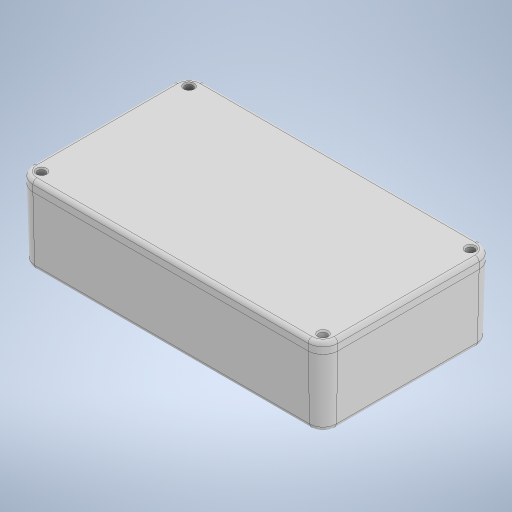
# Autodesk Inventor part: RSpro.Al_DieCast_114x63x30
Saved by Autodesk Inventor 2023 (Build 270158030, 158C)
## iProperties
Created: 2022-11-09
Part Number: RSpro.Al_DieCast_114x63x30
Material: Generic
Document SubType Name: Modeling
Designer: Imogen Heard
Density: 1 g/cm^3
Appearance: Default
Author: Imogen Heard
Autodesk Inventor part; units mm, degrees
ref_plane "YZ Plane" through (0, 0, 0) normal (1, 0, 0) x (0, 1, 0)
ref_plane "XZ Plane" through (0, 0, 0) normal (0, 1, 0) x (-1, 0, 0)
sketch "Sketch1" plane through (0, 0, 0) normal (0, 1, 0) x (-1, 0, 0)
  line L0 (-5, -63.6) -> (-109.5, -63.6)
  line L1 (-114.5, -58.6) -> (-114.5, -5)
  line L2 (-109.5, 0) -> (-5, 0)
  line L3 (0, -5) -> (0, -58.6)
  arc A0 (-5, -63.6) -> (0, -58.6) centre (-5, -58.6) ccw
  arc A1 (-114.5, -58.6) -> (-109.5, -63.6) centre (-109.5, -58.6) ccw
  arc A2 (-109.5, 0) -> (-114.5, -5) centre (-109.5, -5) ccw
  arc A3 (0, -5) -> (-5, 0) centre (-5, -5) ccw
  point P0 (0, 0)
  point P1 (0, 0)
  dimension "d0" = 114.5
  dimension "d1" = 63.6
  dimension "d2" = 5
  constraints: 8 end point, 8 point on circle, 8 tangent, 4 centre point, 3 equal radius, 2 parallel, 2 point on line, 1 coincident, 1 horizontal, 1 perpendicular
  measures "d0" distance between parallel lines of L1 L3
  measures "d1" distance between parallel lines of L0 L2
  measures "d2" radius of A0
extrude "Extrusion1" add sketch "Sketch1" along normal blind 26.3 draft 1.5
sketch "Sketch2" plane through (0, 26.3, 0) normal (0, 1, 0) x (1, 0, 0)
  line L0 (4.8113, 62.7887) -> (109.6887, 62.7887)
  line L1 (113.6887, 58.7887) -> (113.6887, 4.8113)
  line L2 (109.6887, 0.8113) -> (4.8113, 0.8113)
  line L3 (0.8113, 4.8113) -> (0.8113, 58.7887)
  line L4 (115.1887, 58.6) -> (115.1887, 5) projected
  line L5 (109.5, -0.6887) -> (5, -0.6887) projected
  line L6 (5, 64.2887) -> (109.5, 64.2887) projected
  line L7 (-0.6887, 5) -> (-0.6887, 58.6) projected
  arc A0 (4.8113, 62.7887) -> (0.8113, 58.7887) centre (4.8113, 58.7887) ccw
  arc A1 (113.6887, 58.7887) -> (109.6887, 62.7887) centre (109.6887, 58.7887) ccw
  arc A2 (109.6887, 0.8113) -> (113.6887, 4.8113) centre (109.6887, 4.8113) ccw
  arc A3 (0.8113, 4.8113) -> (4.8113, 0.8113) centre (4.8113, 4.8113) ccw
  point P0 (0, 0)
  point P1 (115.1887, 31.8)
  point P2 (57.25, 0.8113)
  dimension "d12" = 1.5
  dimension "d13" = 1.5
  dimension "d14" = 1.5
  dimension "d15" = 1.5
  dimension "d16" = 4
  dimension "d20" = 4
  dimension "d21" = 4
  constraints: 8 end point, 8 point on circle, 8 tangent, 4 centre point, 3 equal radius, 2 midpoint, 2 parallel, 1 horizontal, 1 perpendicular
  measures "d12" distance from line of point (115.189, 31.8) L1
  measures "d13" distance from line of L5 point (57.25, 0.811)
  measures "d14" distance between parallel lines of L6 L0
  measures "d15" distance between parallel lines of L7 L3
  measures "d16" radius of A0
  measures "d20" radius of A3
  measures "d21" radius of A1
ref_plane "Work Plane1" through (0, 1.5, 0) normal (0, -1, 0) x (1, 0, 0)
extrude "Extrusion2" cut sketch "Sketch2" against normal up to surface (24.8 mm away) draft -1.5
sketch "Sketch3" plane through (4.8113, 1.5, -1.4607) normal (0, 1, 0) x (1, 0, 0)
  circle A0 centre (-1.0113, 2.3393) radius 2.65
  circle A1 centre (-1.0113, 58.3393) radius 2.65
  circle A2 centre (105.8887, 2.3393) radius 2.65
  circle A3 centre (105.8887, 58.3393) radius 2.65
  line L0 (-4.8113, 57.1393) -> (-4.8113, 3.5393) projected
  line L1 (0.1887, -1.4607) -> (104.6887, -1.4607) projected
  line L2 (104.6887, 62.1393) -> (0.1887, 62.1393) projected
  line L3 (109.6887, 3.5393) -> (109.6887, 57.1393) projected
  point P0 (-4.8113, -1.4607)
  dimension "d22" = 5.3
  dimension "d23" = 3.8
  dimension "d24" = 3.8
  dimension "d25" = 3.8
  dimension "d26" = 3.8
  constraints: 4 centre point, 3 equal radius, 2 horizontal alignment, 2 vertical alignment
  measures "d22" diameter of A0
  measures "d23" distance from line of L0 A0.centre
  measures "d24" distance from line of L1 A0.centre
  measures "d25" distance from line of L2 A1.centre
  measures "d26" distance from line of L3 A2.centre
extrude "Extrusion3" add sketch "Sketch3" along normal up to surface (24.8 mm away)
fillet "Fillet1" radius 1.5 8 edges at (4.9295, 3.7123, -1.4028) (1.4028, 3.7123, -4.9295) (1.4028, 3.7123, -58.6705) (4.9295, 3.7123, -62.1972) (109.5705, 3.7123, -1.4028) (113.0972, 3.7123, -4.9295) (113.0972, 3.7123, -58.6705) (109.5705, 3.7123, -62.1972)
sketch "Sketch4" plane through (0, 26.3, 0) normal (0, 1, 0) x (1, 0, 0)
  circle A0 centre (3.8, 3.8) radius 1.5
  circle A1 centre (3.8, 59.8) radius 1.5
  circle A2 centre (110.7, 3.8) radius 1.5
  circle A3 centre (110.7, 59.8) radius 1.5
  arc A4 (108.2262, 60.7503) -> (111.6503, 57.3262) centre (110.7, 59.8) ccw projected
  arc A5 (111.6503, 6.2738) -> (108.2262, 2.8497) centre (110.7, 3.8) ccw projected
  arc A6 (2.8497, 57.3262) -> (6.2738, 60.7503) centre (3.8, 59.8) ccw projected
  arc A7 (6.2738, 2.8497) -> (2.8497, 6.2738) centre (3.8, 3.8) ccw projected
  point P0 (0, 0)
  point P1 (111.686, 56.2611)
  point P2 (107.1611, 60.786)
  point P3 (107.1611, 2.814)
  point P4 (111.686, 7.3389)
  point P5 (7.3389, 60.786)
  point P6 (2.814, 56.2611)
  point P7 (2.814, 7.3389)
  point P8 (7.3389, 2.814)
  dimension "d30" = 3
  constraints: 4 centre point, 4 concentric, 3 equal radius
  measures "d30" diameter of A0
fillet "Fillet2" radius 2 8 edges at (113.0355, 0, -62.1355) (57.25, 0, -63.6) (1.4645, 0, -62.1355) (0, 0, -31.8) (1.4645, 0, -1.4645) (57.25, 0, 0) (113.0355, 0, -1.4645) (114.5, 0, -31.8)
hole "Hole1" at (110.7, 26.3, -59.8) at (3.8, 26.3, -59.8) at (3.8, 26.3, -3.8) at (110.7, 26.3, -3.8) direction (0, -1, 0) diameter 2.85 depth 20 tip angle 118 thread size "M3.5x0.6" class "6H" standard "ISO Metric profile"
sketch "Sketch5" plane through (0, 26.3, 0) normal (0, 1, 0) x (1, 0, 0)
  line L0 (4.9813, 64.2887) -> (109.5187, 64.2887)
  line L1 (115.1887, 58.6187) -> (115.1887, 4.9813)
  line L2 (109.5187, -0.6887) -> (4.9813, -0.6887)
  line L3 (-0.6887, 4.9813) -> (-0.6887, 58.6187)
  arc A0 (4.9813, 64.2887) -> (-0.6887, 58.6187) centre (4.9813, 58.6187) ccw
  arc A1 (115.1887, 58.6187) -> (109.5187, 64.2887) centre (109.5187, 58.6187) ccw
  arc A2 (109.5187, -0.6887) -> (115.1887, 4.9813) centre (109.5187, 4.9813) ccw
  arc A3 (-0.6887, 4.9813) -> (4.9813, -0.6887) centre (4.9813, 4.9813) ccw
  point P0 (0, 0)
  point P1 (-0.6887, 64.2887)
  point P2 (115.1887, -0.6887)
  point P3 (-0.6887, -0.6887)
  point P4 (5, 64.2887)
  point P5 (5, -0.6887)
  point P6 (115.1887, 5)
  point P7 (-0.6887, 5)
  dimension "d39" = 5.67
  constraints: 8 end point, 8 point on circle, 8 tangent, 6 point on line, 4 centre point, 3 equal radius, 2 horizontal alignment, 2 parallel, 2 vertical alignment, 1 horizontal, 1 perpendicular
  measures "d39" radius of A0
extrude "Extrusion4" add sketch "Sketch5" along normal blind 4 separate body
fillet "Fillet3" radius 1.5 8 edges at (113.528, 30.3, -0.972) (115.1887, 30.3, -31.8) (113.528, 30.3, -62.628) (57.25, 30.3, -64.2887) (0.972, 30.3, -62.628) (-0.6887, 30.3, -31.8) (0.972, 30.3, -0.972) (57.25, 30.3, 0.6887)
sketch "Sketch6" plane through (0, 30.3, 0) normal (0, 1, 0) x (1, 0, 0)
  circle A0 centre (3.8, 59.8) radius 1.5
  circle A1 centre (110.7, 59.8) radius 1.5
  circle A2 centre (3.8, 3.8) radius 1.5
  circle A3 centre (110.7, 3.8) radius 1.5
  circle A4 centre (3.8, 59.8) radius 1.425 projected
  circle A5 centre (110.7, 59.8) radius 1.425 projected
  circle A6 centre (110.7, 3.8) radius 1.425 projected
  circle A7 centre (3.8, 3.8) radius 1.425 projected
  point P0 (0, 0)
  dimension "d43" = 3
  constraints: 4 centre point, 4 concentric, 3 equal radius
  measures "d43" diameter of A0
hole "Hole2" at (3.8, 30.3, -59.8) at (110.7, 30.3, -59.8) at (110.7, 30.3, -3.8) at (3.8, 30.3, -3.8) direction (0, -1, 0) diameter 3 depth 4 tip angle 118 countersink diameter 4 countersink angle 90 bodies 2
sketch "Sketch7" plane through (0, 26.3, 0) normal (0, -1, 0) x (1, 0, 0)
  line L0 (113.1887, -10.8113) -> (113.1887, -52.7887)
  line L1 (103.6887, -62.2887) -> (10.8113, -62.2887)
  line L2 (1.3113, -52.7887) -> (1.3113, -10.8113)
  line L3 (10.8113, -2.3113) -> (103.6887, -2.3113)
  line L4 (111.6887, -10.8113) -> (111.6887, -52.7887)
  line L5 (103.6887, -61.2887) -> (10.8113, -61.2887)
  line L6 (2.3113, -52.7887) -> (2.3113, -10.8113)
  line L7 (106.8264, -0.8113) -> (7.6736, -0.8113) projected
  line L8 (7.6736, -62.7887) -> (106.8264, -62.7887) projected
  line L9 (0.8113, -7.6736) -> (0.8113, -55.9264) projected
  line L10 (113.6887, -55.9264) -> (113.6887, -7.6736) projected
  arc A0 (108.2262, -2.8497) -> (111.6503, -6.2738) centre (110.7, -3.8) ccw projected
  line L11 (10.8113, -1.3113) -> (103.6887, -1.3113)
  line L12 (113.1887, -10.8113) -> (111.6887, -10.8113)
  line L13 (103.6887, -2.3113) -> (103.6887, -1.3113)
  line L14 (103.6887, -62.2887) -> (103.6887, -61.2887)
  line L15 (111.6887, -52.7887) -> (113.6887, -52.7887)
  line L16 (10.8113, -61.2887) -> (10.8113, -62.2887)
  line L17 (10.8113, -1.3113) -> (10.8113, -2.3113)
  line L18 (2.3113, -10.8113) -> (1.3113, -10.8113)
  line L19 (1.3113, -52.7887) -> (2.3113, -52.7887)
  point P0 (0, 0)
  point P1 (103.6887, -52.7887)
  point P2 (7.8641, -10.8113)
  point P3 (103.6887, -1.8113)
  point P4 (1.8113, -52.7887)
  point P5 (112.6887, -52.7887)
  point P6 (10.8113, -1.8113)
  point P7 (10.8113, -61.7887)
  point P8 (7.8641, -62.1393)
  point P9 (103.6887, -61.7887)
  point P10 (1.8113, -10.8113)
  point P11 (112.4387, -10.8113)
  dimension "d52" = 0.5
  dimension "d53" = 0.5
  dimension "d54" = 0.5
  dimension "d55" = 1.5
  dimension "d56" = 1.5
  dimension "d57" = 1.5
  dimension "d58" = 1.5
  dimension "d60" = 0.5
  dimension "d62" = 10
  dimension "d63" = 10
  dimension "d64" = 10
  dimension "d65" = 10
  constraints: 32 end point, 8 midpoint, 5 horizontal alignment, 4 parallel, 4 vertical alignment, 2 horizontal, 2 perpendicular, 2 point on line
  measures "d52" distance between parallel lines of L8 L1
  measures "d53" distance between parallel lines of L9 L2
  measures "d54" distance between parallel lines of L10 L0
  measures "d55" distance between parallel lines of L0 L4
  measures "d56" distance between parallel lines of L7 L3
  measures "d57" distance between parallel lines of L6 L9
  measures "d58" distance between parallel lines of L5 L8
  measures "d60" distance between parallel lines of L11 L7
  measures "d62" distance between parallel lines of L7 L12
  measures "d63" distance between parallel lines of L10 L13
  measures "d64" distance between parallel lines of L8 L15
  measures "d65" distance between parallel lines of L9 L16
extrude "Extrusion5" add sketch "Sketch7" along normal blind 2.5 bodies 2
sketch "Sketch8" plane through (0, 26.3, 0) normal (0, -1, 0) x (1, 0, 0)
  line L0 (10.8113, -2.3113) -> (103.6887, -2.3113)
  line L1 (111.6887, -10.8113) -> (111.6887, -52.7887)
  line L2 (103.6887, -61.2887) -> (10.8113, -61.2887)
  line L3 (2.3113, -52.7887) -> (2.3113, -10.8113)
  line L4 (2.3113, -10.8113) -> (1.3113, -10.8113) projected
  arc A0 (2.3113, -10.8113) -> (10.8113, -2.3113) centre (1.8245, -1.8245) ccw
  arc A1 (111.6887, -52.7887) -> (103.6887, -61.2887) centre (112.6777, -61.7342) ccw
  arc A2 (103.6887, -2.3113) -> (111.6887, -10.8113) centre (112.6777, -1.8658) ccw
  arc A3 (10.8113, -61.2887) -> (2.3113, -52.7887) centre (1.8245, -61.7755) ccw
  line L5 (1.3113, -10.8113) -> (1.3113, -52.7887) projected
  point P0 (2.3113, -2.3113)
  point P1 (111.6887, -61.2887)
  point P2 (111.6887, -2.3113)
  point P3 (103.6887, -2.3113)
  point P4 (111.6887, -10.8113)
  dimension "d71" = 9
  dimension "d72" = 9
  dimension "d73" = 9
  dimension "d74" = 9
  dimension "d75" = 1
  constraints: 13 point on circle, 8 end point, 4 centre point, 3 coincident, 2 horizontal alignment, 2 parallel, 2 vertical alignment, 1 horizontal, 1 perpendicular
  measures "d71" radius of A0
  measures "d72" radius of A2
  measures "d73" radius of A1
  measures "d74" radius of A3
  measures "d75" distance between parallel lines of L5 L3
extrude "Extrusion6" cut sketch "Sketch8" against normal blind 2.5 bodies 2
equation "\"d23\" = d24"
equation "\"d25\" = d24"
equation "\"d26\" = d23"
equation "\"d64\" = d62"
equation "\"d65\" = d62"
